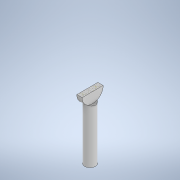
# Autodesk Inventor part: штырь
Saved by Autodesk Inventor 2022 (Build 260153000, 153)
## iProperties
Created: 2024-04-28
Part Number: штырь
Material: Типовые
Document SubType Name: Modeling
Designer: Pavel
Density: 1 g/cm^3
Appearance: По умолчанию
Mass: 0.0094674 g
Surface Area: 0.424301 cm^2
Volume: 0.0094674 cm^3
Author: Pavel
Autodesk Inventor part; units mm, degrees
ref_plane "YZ Plane" through (0, 0, 0) normal (1, 0, 0) x (0, 1, 0)
ref_plane "XZ Plane" through (0, 0, 0) normal (0, 1, 0) x (-1, 0, 0)
sketch "Эскиз1" plane through (0, 0, 0) normal (0, 1, 0) x (-1, 0, 0)
  circle A0 centre (0, 0) radius 0.5
  dimension "d0" = 1
  constraints: 1 centre point, 1 coincident
  measures "d0" diameter of A0
extrude "Выдавливание1" add sketch "Эскиз1" along normal blind 12
sketch "Эскиз2" plane through (0, 0, 0) normal (1, 0, 0) x (0, 1, 0)
  line L0 (0, 0) -> (6, 0) construction
  circle A0 centre (6, 0) radius 1
  dimension "d3" = 6
  dimension "d4" = 2
  constraints: 2 end point, 1 centre point, 1 coincident, 1 horizontal
  measures "d3" distance of L0.start L0.end
  measures "d4" diameter of A0
extrude "Выдавливание2" add sketch "Эскиз2" along normal mid plane 0.5
sketch "Эскиз3" plane through (-0.25, 0, 0) normal (-1, 0, 0) x (0, 0, 1)
  line L0 (0, 0) -> (0, 6) construction
  circle A0 centre (0, 6) radius 1
  dimension "d7" = 6
  dimension "d8" = 2
  constraints: 2 end point, 1 centre point, 1 coincident, 1 vertical
  measures "d7" distance of L0.start L0.end
  measures "d8" diameter of A0
extrude "Выдавливание3" cut sketch "Эскиз3" along normal blind 1.25
sketch "Эскиз4" plane through (-0.25, 0, 0) normal (-1, 0, 0) x (0, 0, 1)
  point P0 (0, 0)
ref_plane "РабПлоскость1" through (0, 0, 0) normal (-1, 0, 0) x (0, 0, 1)
sketch "Эскиз6" plane through (0.25, 0, 0) normal (1, 0, 0) x (0, 0, -1)
  circle A0 centre (0, 6) radius 1
  point P0 (0, 0)
  constraints: 1 centre point
extrude "Выдавливание5" cut sketch "Эскиз6" along normal blind 3
